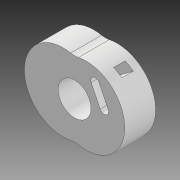
# Autodesk Inventor part: TestRotor
Saved by Autodesk Inventor 2020 (Build 240168000, 168)
## iProperties
Created: 2021-05-17
Part Number: TestRotor
Material: Generic
Document SubType Name: Modeling
Designer: DDeGo
Density: 1 g/cm^3
Appearance: Default
Author: DDeGo
Autodesk Inventor part; units mm, degrees
ref_plane "YZ Plane" through (0, 0, 0) normal (1, 0, 0) x (0, 1, 0)
ref_plane "XZ Plane" through (0, 0, 0) normal (0, 1, 0) x (-1, 0, 0)
ref_plane "XY Plane" through (0, 0, 0) normal (0, 0, 1) x (1, 0, 0)
sketch "Sketch1" plane through (0, 0, 0) normal (0, 0, 1) x (1, 0, 0)
  arc A0 (-0.7987, -9.9681) -> (-0.7987, 9.9681) centre (0, 0) ccw
  arc A1 (-4.2013, 9.9681) -> (-4.2013, -9.9681) centre (-5, 0) ccw
  line L0 (-5, 0) -> (0, 0) construction
  arc A2 (-4.2013, 9.9681) -> (-0.7987, 9.9681) centre (-2.5, 31.2) ccw
  arc A3 (-0.7987, -9.9681) -> (-4.2013, -9.9681) centre (-2.5, -31.2) ccw
  circle A4 centre (-2.5, 0) radius 5
  line L1 (-15, 10) -> (10, 10) construction
  line L2 (10, 10) -> (10, -10) construction
  line L3 (10, -10) -> (-15, -10) construction
  line L4 (-15, -10) -> (-15, 10) construction
  dimension "d0" = 5
  dimension "d2" = 10
  dimension "d4" = 10
  dimension "d13" = 25
  dimension "d14" = 0.1
  constraints: 10 end point, 8 point on circle, 8 tangent, 5 centre point, 2 equal radius, 2 horizontal, 2 parallel, 1 coincident, 1 midpoint, 1 perpendicular
  measures "d0" distance of L0.start L0.end
  measures "d2" radius of A1
  measures "d4" diameter of A4
  measures "d13" distance between parallel lines of L2 L4
  measures "d14" distance edge to line of A2 L1
extrude "Extrusion1" add sketch "Sketch1" along normal blind 8
sketch "Sketch3" plane through (0, 0, 8) normal (0, 0, 1) x (1, 0, 0)
  line L0 (3.397, 1.9529) -> (2.603, 6.0471) construction
  line L1 (2.7436, 1.8262) -> (1.9495, 5.9204)
  line L2 (3.2564, 6.1738) -> (4.0505, 2.0796)
  arc A0 (2.7436, 1.8262) -> (4.0505, 2.0796) centre (3.397, 1.9529) ccw
  arc A1 (3.2564, 6.1738) -> (1.9495, 5.9204) centre (2.603, 6.0471) ccw
  point P0 (0, 0)
  point P1 (3, 4)
  dimension "d17" = 4
  dimension "d18" = 3
  constraints: 8 end point, 4 point on circle, 4 tangent, 2 centre point, 1 midpoint, 1 parallel
  measures "d17" vertical distance of point (0, 0) point (3, 4)
  measures "d18" horizontal distance of point (3, 4) point (0, 0)
extrude "Extrusion3" cut sketch "Sketch3" against normal blind 3
sketch "Sketch4" plane through (0, 0, 5) normal (0, 0, 1) x (1, 0, 0)
  arc A0 (3.2564, 6.1738) -> (1.9495, 5.9204) centre (2.603, 6.0471) ccw projected
  line L0 (2.603, 6.0471) -> (6.341, 8.844) construction
  line L1 (3.2872, 5.1326) -> (7.0252, 7.9295)
  line L2 (5.6568, 9.7584) -> (1.9188, 6.9616)
  arc A1 (1.9188, 6.9616) -> (3.2872, 5.1326) centre (2.603, 6.0471) ccw
  arc A2 (7.0252, 7.9295) -> (5.6568, 9.7584) centre (6.341, 8.844) ccw
  point P0 (0, 0)
  point P1 (4.472, 7.4455)
  point P2 (1.2962, 5.8498)
  constraints: 8 end point, 4 point on circle, 4 tangent, 2 centre point, 1 midpoint, 1 parallel, 1 other
extrude "Extrusion4" cut sketch "Sketch4" against normal blind 3
sketch "Sketch5" plane through (0, 0, 8) normal (0, 0, 1) x (1, 0, 0)
  line L0 (-11.2717, 11.7043) -> (-7.2775, 7.7101)
  line L1 (-7.2775, 7.7101) -> (-8.4228, 6.5648)
  line L2 (-8.4228, 6.5648) -> (-12.417, 10.559)
  line L3 (-12.417, 10.559) -> (-11.2717, 11.7043)
  point P0 (0, 0)
  constraints: 8 end point, 2 parallel, 1 perpendicular
extrude "Extrusion5" cut sketch "Sketch5" against normal blind 1
pattern_circular "Circular Pattern1" count 2 over 360 about axis through (-2.5, 0, 0) along (0, 0, 1) of "Extrusion3", "Extrusion4", "Extrusion5"
body "Solid1"
